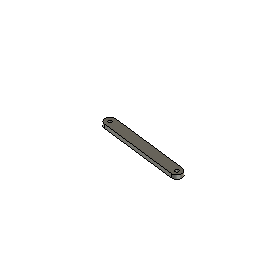
arm_half (Autodesk Fusion 360 design; units mm, degrees)
Autodesk Fusion 360 part; units mm, degrees
sketch "Sketch1" plane through (0, 0, -11.43) normal (0, 0, -1) x (1, 0, 0)
  circle A0 centre (0, -44.0795) radius 1.5875
  line L0 (-7.4959, -38.9995) -> (-7.4959, -49.1595)
  line L1 (-7.4959, -49.1595) -> (7.4959, -49.1595)
  line L2 (7.4959, -49.1595) -> (7.4959, -38.9995)
  line L3 (7.4959, -38.9995) -> (-7.4959, -38.9995)
  circle A1 centre (0, -44.0795) radius 1.5875
  line L4 (0, -44.0795) -> (76.2, -44.0795) construction
  circle A2 centre (76.2, -44.0795) radius 1.5875
  line L5 (0, -49.1595) -> (76.2, -49.1595)
  arc A3 (76.2, -49.1595) -> (76.2, -38.9995) centre (76.2, -44.0795) ccw
  line L6 (76.2, -38.9995) -> (0, -38.9995)
  arc A4 (0, -38.9995) -> (0, -49.1595) centre (0, -44.0795) ccw
  line L7 (0, -44.0795) -> (76.2, -44.0795) construction
  dimension "d281" = 76.2
  dimension "d282" = 3.175
  dimension "d283" = 10.16
  constraint coincident A0.centre A1.centre
  constraint horizontal L4
  constraint coincident L4.end A2.centre
  constraint tangent L5 A3
  constraint tangent A3 L6
  constraint parallel L5 L6
  constraint tangent L6 A4
  constraint tangent L5 A4
  constraint perpendicular L2 L7
  measures "d281" distance of A0.centre L4.end
  measures "d282" diameter of A2
  measures "d283" diameter of A3
extrude "Extrude1" add sketch "Sketch1" along normal blind 3.81 contours L1 L2 L3 L5 L6 A4 | L2 L5 A3 L6 in component "Component"
component "Component" placed x (0.992427, -0.122837, 0) y (0.122837, 0.992427, 0) z (0, 0, 1) at (-7.0021, 0.3338, 0)
